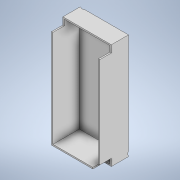
# Autodesk Inventor part: brainholder
Saved by Autodesk Inventor 2022 (Build 260153000, 153)
## iProperties
Created: 2021-01-11
Part Number: brainholder
Material: Generic
Document SubType Name: Modeling
Designer: papa
Density: 1 g/cm^3
Appearance: Default
Author: papa
Autodesk Inventor part; units mm, degrees
ref_plane "YZ Plane" through (0, 0, 0) normal (1, 0, 0) x (0, 1, 0)
ref_plane "XZ Plane" through (0, 0, 0) normal (0, 1, 0) x (-1, 0, 0)
ref_plane "XY Plane" through (0, 0, 0) normal (0, 0, 1) x (1, 0, 0)
sketch "Sketch1" plane through (0, 0, 0) normal (0, 0, 1) x (1, 0, 0)
  line L0 (0, 0) -> (34, 0)
  line L1 (34, 0) -> (34, 74)
  line L2 (34, 74) -> (0, 74)
  line L3 (0, 74) -> (0, 0)
  line L4 (33, 73) -> (1, 73)
  line L5 (1, 73) -> (1, 1)
  line L6 (1, 1) -> (33, 1)
  line L7 (33, 1) -> (33, 73)
  dimension "d0" = 34
  dimension "d1" = 74
  dimension "d2" = 1
  dimension "d3" = 1
  dimension "d4" = 1
  dimension "d5" = 1
  constraints: 16 end point, 4 parallel, 2 horizontal, 2 perpendicular
  measures "d0" distance of L2.end L1.end
  measures "d1" distance of L1.end L0.end
  measures "d2" distance between parallel lines of L3 L5
  measures "d3" distance between parallel lines of L0 L6
  measures "d4" distance between parallel lines of L1 L7
  measures "d5" distance between parallel lines of L2 L4
extrude "Extrusion1" add sketch "Sketch1" along normal blind 1.5 contours L3 L2 L1 L0 | L7 L6 L5 L4
extrude "Extrusion2" add sketch "Sketch1" along normal blind 20
sketch "Sketch2" plane through (0, 0, 0) normal (0, 0, -1) x (-1, 0, 0)
  circle A0 centre (-32, 2) radius 1
  circle A1 centre (-2, 72) radius 1
  line L0 (0, 74) -> (0, 0) projected
  line L1 (-34, 74) -> (0, 74) projected
  line L2 (0, 0) -> (-34, 0) projected
  line L3 (-34, 0) -> (-34, 74) projected
  dimension "d10" = 2
  dimension "d11" = 2
  dimension "d12" = 2
  dimension "d13" = 2
  dimension "d14" = 2
  dimension "d15" = 2
  constraints: 2 centre point
  measures "d10" diameter of A0
  measures "d11" diameter of A1
  measures "d12" distance from line of L0 A1.centre
  measures "d13" distance from line of L1 A1.centre
  measures "d14" distance from line of L2 A0.centre
  measures "d15" distance from line of L3 A0.centre
extrude "Extrusion3" cut sketch "Sketch2" against normal through all contours A0 | A1
sketch "Sketch3" plane through (0, 0, 20) normal (0, 0, 1) x (1, 0, 0)
  line L0 (34, 74) -> (0, 74) projected
  line L1 (34, 0) -> (34, 74) projected
  line L2 (0, 74) -> (34, 74)
  line L3 (34, 74) -> (34, 69)
  line L4 (34, 69) -> (0, 69)
  line L5 (0, 69) -> (0, 74)
  line L6 (34, 0) -> (29, 0)
  line L7 (29, 0) -> (29, 5)
  line L8 (29, 5) -> (34, 5)
  line L9 (34, 5) -> (34, 0)
  point P0 (0, 0)
  dimension "d20" = 5
  dimension "d21" = 5
  dimension "d22" = 5
  constraints: 16 end point, 4 parallel, 2 horizontal, 2 perpendicular, 1 point on line
  measures "d20" distance of L7.end L8.end
  measures "d21" distance of L6.end L7.end
  measures "d22" distance between parallel lines of L4 L0
extrude "Extrusion4" cut sketch "Sketch3" against normal blind 8
chamfer "Chamfer1" distance 1.5 angle 45 2 edges at (3, 72, 0) (33, 2, 0)
body "Solid1"
